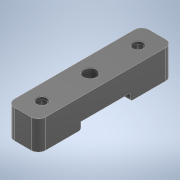
# Autodesk Inventor part: Base
Saved by Autodesk Inventor 2022 (Build 260153000, 153)
## iProperties
Created: 2021-11-22
Part Number: Base
Material: Genérico
Document SubType Name: Modeling
Designer: JK
Density: 1 g/cm^3
Appearance: Suave - Negro
Author: JK
Autodesk Inventor part; units mm, degrees
ref_plane "YZ Plane" through (0, 0, 0) normal (1, 0, 0) x (0, 1, 0)
ref_plane "XZ Plane" through (0, 0, 0) normal (0, 1, 0) x (-1, 0, 0)
ref_plane "XY Plane" through (0, 0, 0) normal (0, 0, 1) x (1, 0, 0)
sketch "Boceto1" plane through (0, 0, 0) normal (0, 1, 0) x (-1, 0, 0)
  line L0 (-6.5, 28) -> (6.5, 28)
  line L1 (6.5, 28) -> (6.5, -28)
  line L2 (6.5, -28) -> (-6.5, -28)
  line L3 (-6.5, -28) -> (-6.5, 28)
  line L4 (-6.5, 28) -> (6.5, -28) construction
  line L5 (6.5, 28) -> (-6.5, -28) construction
  line L6 (5.15, 26.15) -> (-5.15, 26.15)
  line L7 (-5.15, 26.15) -> (-5.15, 13.85)
  line L8 (-5.15, 13.85) -> (5.15, 13.85)
  line L9 (5.15, 13.85) -> (5.15, 26.15)
  line L10 (5.15, 26.15) -> (-5.15, 13.85) construction
  line L11 (-5.15, 26.15) -> (5.15, 13.85) construction
  line L12 (5.15, -13.85) -> (-5.15, -13.85)
  line L13 (-5.15, -13.85) -> (-5.15, -26.15)
  line L14 (-5.15, -26.15) -> (5.15, -26.15)
  line L15 (5.15, -26.15) -> (5.15, -13.85)
  line L16 (5.15, -13.85) -> (-5.15, -26.15) construction
  line L17 (-5.15, -13.85) -> (5.15, -26.15) construction
  point P0 (0, 0)
  point P1 (0, 20)
  point P2 (0, -20)
  point P3 (0, 20)
  point P4 (0, 0)
  point P5 (0, -20)
  point P6 (0, 0)
  dimension "d0" = 12.3
  dimension "d1" = 10.3
  dimension "d2" = 20
  dimension "d3" = 56
  dimension "d4" = 20
  dimension "d5" = 13
  constraints: 36 end point, 10 midpoint, 6 parallel, 3 horizontal, 3 perpendicular, 2 equal length, 2 vertical alignment
  measures "d0" distance of L8.end L6.start
  measures "d1" distance of L7.end L8.end
  measures "d2" distance of point (0, 0) point (0, 20)
  measures "d3" distance of L0.end L1.end
  measures "d4" distance of point (0, 0) point (0, -20)
  measures "d5" distance of L1.end L2.end
extrude "Extrusión1" add sketch "Boceto1" along normal blind 15
sketch "Boceto2" plane through (0, 15, 0) normal (0, 1, 0) x (1, 0, 0)
  line L0 (6.5, 28) -> (-6.5, 28) projected
  line L1 (-6.5, 28) -> (-6.5, -28) projected
  line L2 (-6.5, -28) -> (6.5, -28) projected
  line L3 (6.5, -28) -> (6.5, 28) projected
  line L4 (-5.15, -26.15) -> (-5.15, -13.85) projected
  line L5 (-5.15, -13.85) -> (5.15, -13.85) projected
  line L6 (5.15, -13.85) -> (5.15, -26.15) projected
  line L7 (5.15, -26.15) -> (-5.15, -26.15) projected
  line L8 (-5.15, 13.85) -> (-5.15, 26.15) projected
  line L9 (-5.15, 26.15) -> (5.15, 26.15) projected
  line L10 (5.15, 26.15) -> (5.15, 13.85) projected
  line L11 (5.15, 13.85) -> (-5.15, 13.85) projected
  point P0 (0, 0)
extrude "Extrusión2" add sketch "Boceto2" along normal blind 1 contours L3 L2 L1 L0 | L4 L5 L6 L7 | L8 L9 L10 L11
sketch "Boceto3" plane through (0, 0, 0) normal (0, -1, 0) x (1, 0, 0)
  circle A0 centre (0, 20) radius 2.15
  circle A1 centre (0, -20) radius 2.15
  line L0 (-5.15, 13.85) -> (5.15, 13.85) projected
  line L1 (5.15, -13.85) -> (-5.15, -13.85) projected
  line L2 (5.15, 13.85) -> (5.15, 26.15) projected
  point P0 (0, 0)
  dimension "d10" = 4.3
  dimension "d11" = 6.15
  dimension "d12" = 6.15
  dimension "d13" = 5.15
  constraints: 2 centre point, 1 equal radius, 1 vertical alignment
  measures "d10" diameter of A0
  measures "d11" distance from line of L0 A0.centre
  measures "d12" distance from line of L1 A1.centre
  measures "d13" distance from line of L2 A0.centre
extrude "Extrusión3" cut sketch "Boceto3" against normal through all
fillet "Empalme1" radius 1.15 8 edges at (5.15, 7.5, -13.85) (5.15, 7.5, 26.15) (5.15, 7.5, 13.85) (5.15, 7.5, -26.15) (-5.15, 7.5, -26.15) (-5.15, 7.5, 13.85) (-5.15, 7.5, -13.85) (-5.15, 7.5, 26.15)
fillet "Empalme2" radius 3 4 edges at (6.5, 8, -28) (6.5, 8, 28) (-6.5, 8, 28) (-6.5, 8, -28)
sketch "Boceto6" plane through (-6.5, 0, -25) normal (-1, 0, 0) x (0, 0, 1)
  line L0 (35.25, -7) -> (14.75, -7)
  line L1 (14.75, -7) -> (14.75, 7)
  line L2 (14.75, 7) -> (35.25, 7)
  line L3 (35.25, 7) -> (35.25, -7)
  line L4 (35.25, -7) -> (14.75, 7) construction
  line L5 (14.75, -7) -> (35.25, 7) construction
  point P0 (25, 0)
  dimension "d30" = 20.5
  dimension "d31" = 7
  constraints: 12 end point, 2 midpoint, 2 parallel, 1 horizontal, 1 perpendicular
  measures "d30" distance between parallel lines of L3 L1
  measures "d31" distance from line of L2 point (25, 0)
extrude "Extrusión6" cut sketch "Boceto6" against normal through all
sketch "Boceto7" plane through (0, 16, 0) normal (0, 1, 0) x (1, 0, 0)
  circle A0 centre (0, 0) radius 2.7
  dimension "d35" = 5.4
  constraints: 1 centre point, 1 coincident
  measures "d35" diameter of A0
extrude "Extrusión7" cut sketch "Boceto7" against normal through all
sketch "Boceto8" plane through (0, 0, 0) normal (0, -1, 0) x (1, 0, 0)
  line L0 (4, -13.85) -> (-4, -13.85) projected
  arc A0 (5.15, -15) -> (4, -13.85) centre (4, -15) ccw projected
  line L1 (5.15, -25) -> (5.15, -15) projected
  arc A1 (4, -26.15) -> (5.15, -25) centre (4, -25) ccw projected
  line L2 (-4, -26.15) -> (4, -26.15) projected
  arc A2 (-5.15, -25) -> (-4, -26.15) centre (-4, -25) ccw projected
  line L3 (-5.15, -15) -> (-5.15, -25) projected
  arc A3 (-4, -13.85) -> (-5.15, -15) centre (-4, -15) ccw projected
  line L4 (6.5, -10.25) -> (-6.5, -10.25) projected
  line L5 (-6.5, -25) -> (-6.5, -10.25) projected
  arc A4 (-6.5, -25) -> (-3.5, -28) centre (-3.5, -25) ccw projected
  line L6 (3.5, -28) -> (-3.5, -28) projected
  arc A5 (3.5, -28) -> (6.5, -25) centre (3.5, -25) ccw projected
  line L7 (6.5, -10.25) -> (6.5, -25) projected
  line L8 (-6.5, 10.25) -> (6.5, 10.25) projected
  line L9 (6.5, 25) -> (6.5, 10.25) projected
  arc A6 (6.5, 25) -> (3.5, 28) centre (3.5, 25) ccw projected
  line L10 (-3.5, 28) -> (3.5, 28) projected
  arc A7 (-3.5, 28) -> (-6.5, 25) centre (-3.5, 25) ccw projected
  line L11 (-6.5, 10.25) -> (-6.5, 25) projected
  line L12 (4, 26.15) -> (-4, 26.15) projected
  arc A8 (5.15, 25) -> (4, 26.15) centre (4, 25) ccw projected
  line L13 (5.15, 15) -> (5.15, 25) projected
  arc A9 (4, 13.85) -> (5.15, 15) centre (4, 15) ccw projected
  line L14 (-4, 13.85) -> (4, 13.85) projected
  arc A10 (-5.15, 15) -> (-4, 13.85) centre (-4, 15) ccw projected
  line L15 (-5.15, 25) -> (-5.15, 15) projected
  arc A11 (-4, 26.15) -> (-5.15, 25) centre (-4, 25) ccw projected
  point P0 (0, 0)
extrude "Extrusión8" cut sketch "Boceto8" against normal blind 4
fillet "Empalme5" radius 1 2 edges at (0, 4, -10.25) (0, 4, 10.25)
sketch "Boceto4" plane through (0, 16, 0) normal (0, 1, 0) x (1, 0, 0)
  circle A0 centre (0, -5) radius 1.7
  circle A1 centre (0, 5) radius 1.7
  point P0 (0, 0)
  dimension "d19" = 3.4
  dimension "d25" = 5
  dimension "d26" = 5
  constraints: 2 centre point, 1 equal radius
  measures "d19" diameter of A0
  measures "d25" distance of A1.centre point (0, 0)
  measures "d26" distance of point (0, 0) A0.centre
sketch "Boceto5" plane through (0, 0, 0) normal (0, -1, 0) x (1, 0, 0)
  circle A0 centre (0, 5) radius 1.7 projected
  circle A1 centre (0, 5) radius 2.8
  circle A2 centre (0, -5) radius 1.7 projected
  circle A3 centre (0, -5) radius 2.8
  line L0 (3.2332, 5) -> (1.6166, 2.2)
  line L1 (1.6166, 2.2) -> (-1.6166, 2.2)
  line L2 (-1.6166, 2.2) -> (-3.2332, 5)
  line L3 (-3.2332, 5) -> (-1.6166, 7.8)
  line L4 (-1.6166, 7.8) -> (1.6166, 7.8)
  line L5 (1.6166, 7.8) -> (3.2332, 5)
  line L6 (3.2332, -5) -> (1.6166, -7.8)
  line L7 (1.6166, -7.8) -> (-1.6166, -7.8)
  line L8 (-1.6166, -7.8) -> (-3.2332, -5)
  line L9 (-3.2332, -5) -> (-1.6166, -2.2)
  line L10 (-1.6166, -2.2) -> (1.6166, -2.2)
  line L11 (1.6166, -2.2) -> (3.2332, -5)
  point P0 (0, 0)
  dimension "d27" = 5.6
  constraints: 24 end point, 4 coincident, 2 centre point, 2 horizontal alignment, 2 tangent, 1 equal radius, 26 other
  measures "d27" diameter of A1
equation "\"d4\" = d2"
